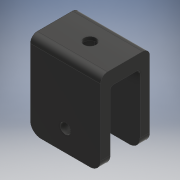
# Autodesk Inventor part: X_Idler
Saved by Autodesk Inventor 2017.3 (Build 213256000, 256)
## iProperties
Created: 2018-09-09
Part Number: X_Idler
Material: ABS Plastic
Document SubType Name: Modeling
Designer: Ax
Density: 1.06 g/cm^3
Appearance: Smooth - Black
Author: Ax
## iProperties of the stored document X_Idler_3DPrint.ipt
Created: 2018-09-09
Part Number: X_Idler_3DPrint
Material: Generic
Document SubType Name: Modeling
Designer: Ax
Density: 1 g/cm^3
Appearance: Default
Author: Ax
Autodesk Inventor part; units mm, degrees
ref_plane "YZ Plane" through (0, 0, 0) normal (1, 0, 0) x (0, 1, 0)
ref_plane "XZ Plane" through (0, 0, 0) normal (0, 1, 0) x (-1, 0, 0)
ref_plane "XY Plane" through (0, 0, 0) normal (0, 0, 1) x (1, 0, 0)
sketch "Sketch1" plane through (0, 0, 0) normal (1, 0, 0) x (0, 1, 0)
  line L0 (7, -20) -> (7, 4)
  line L1 (7, 4) -> (-7, 4)
  line L2 (-7, 4) -> (-7, -20)
  line L3 (-7, -20) -> (-4.25, -20)
  line L4 (-4.25, -20) -> (-4.25, 0)
  line L5 (-4.25, 0) -> (4.25, 0)
  line L6 (4.25, 0) -> (4.25, -20)
  line L7 (4.25, -20) -> (7, -20)
  line L8 (0, 0) -> (0, 4) construction
  dimension "d0" = 8.5
  dimension "d1" = 24
  dimension "d2" = 4
  dimension "d4" = 14
  constraints: 18 end point, 6 perpendicular, 2 equal length, 2 midpoint, 2 vertical, 1 coincident, 1 symmetric about line
  measures "d0" distance of L4.end L5.end
  measures "d1" distance of L0.start L0.end
  measures "d2" vertical distance of L0.end L5.end
  measures "d4" distance of L2.end L0.start
extrude "Extrusion1" add sketch "Sketch1" along normal mid plane 20
sketch "Sketch2" plane through (-10, 7, 4) normal (0, 1, 0) x (1, 0, 0)
  line L0 (10, 24) -> (10, 0) construction
  line L1 (20, 24) -> (0, 24) construction
  line L2 (0, 0) -> (20, 0) construction
  circle A0 centre (10, 18) radius 1.5
  point P0 (10, 4)
  dimension "d7" = 3
  dimension "d8" = 6
  constraints: 2 end point, 2 midpoint, 1 centre point, 1 point on line, 1 vertical
  measures "d7" diameter of A0
  measures "d8" distance of L0.start A0.centre
extrude "Extrusion2" cut sketch "Sketch2" against normal through all
sketch "Sketch3" plane through (-10, -7, 4) normal (0, 0, 1) x (1, 0, 0)
  circle A0 centre (10, 7) radius 1.7
  dimension "d11" = 3.4
  constraints: 1 centre point, 1 coincident
  measures "d11" diameter of A0
extrude "Extrusion3" cut sketch "Sketch3" against normal up to surface (4 mm away)
sketch "Sketch4" plane through (10, 4.25, 0) normal (0, 0, -1) x (-1, 0, 0)
  line L0 (13.2909, -4.25) -> (11.6454, -7.1)
  line L1 (11.6454, -7.1) -> (8.3546, -7.1)
  line L2 (8.3546, -7.1) -> (6.7091, -4.25)
  line L3 (6.7091, -4.25) -> (8.3546, -1.4)
  line L4 (8.3546, -1.4) -> (11.6454, -1.4)
  line L5 (11.6454, -1.4) -> (13.2909, -4.25)
  point P0 (10, -4.25)
  point P1 (10, -4.25)
  dimension "d14" = 5.7
  constraints: 12 end point, 1 coincident, 1 horizontal, 13 other
  measures "d14" distance of L4.end L0.end
extrude "Extrusion4" cut sketch "Sketch4" against normal blind 3
fillet "Fillet1" radius 2 2 edges at (0, 7, 4) (0, -7, 4)
fillet "Fillet2" radius 3 4 edges at (10, -5.625, -20) (10, 5.625, -20) (-10, 5.625, -20) (-10, -5.625, -20)
fillet "Fillet3" radius 1 2 edges at (0, 4.25, 0) (0, -4.25, 0)
body "Solid1"
